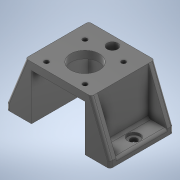
# Autodesk Inventor part: zmotorsupport
Saved by Autodesk Inventor 2020.2 (Build 242310000, 310)
## iProperties
Created: 2020-07-31
Part Number: zmotorsupport
Material: Generic
Document SubType Name: Modeling
Designer: JK
Density: 1 g/cm^3
Appearance: Smooth - Black
Author: JK
Autodesk Inventor part; units mm, degrees
ref_plane "YZ Plane" through (0, 0, 0) normal (1, 0, 0) x (0, 1, 0)
ref_plane "XZ Plane" through (0, 0, 0) normal (0, 1, 0) x (-1, 0, 0)
ref_plane "XY Plane" through (0, 0, 0) normal (0, 0, 1) x (1, 0, 0)
sketch "Sketch1" plane through (0, 0, 0) normal (0, 1, 0) x (-1, 0, 0)
  circle A0 centre (0, 0) radius 11.5
  circle A1 centre (0, -22) radius 4.25
  line L0 (-21.5, 21.5) -> (21.5, 21.5)
  line L1 (21.5, 21.5) -> (21.5, -21.5)
  line L2 (21.5, -21.5) -> (-21.5, -21.5)
  line L3 (-21.5, -21.5) -> (-21.5, 21.5)
  line L4 (-21.5, 21.5) -> (21.5, -21.5) construction
  line L5 (21.5, 21.5) -> (-21.5, -21.5) construction
  line L6 (21.5, -21.5) -> (-21.5, -21.5)
  line L7 (-21.5, -21.5) -> (-21.5, -29.5)
  line L8 (-21.5, -29.5) -> (21.5, -29.5)
  line L9 (21.5, -29.5) -> (21.5, -21.5)
  circle A2 centre (15.5, 15.5) radius 1.8
  circle A3 centre (15.5, -15.5) radius 1.8
  circle A4 centre (-15.5, -15.5) radius 1.8
  circle A5 centre (-15.5, 15.5) radius 1.8
  point P0 (0, 0)
  dimension "d0" = 23
  dimension "d1" = 22
  dimension "d2" = 8.5
  dimension "d3" = 43
  dimension "d4" = 43
  dimension "d5" = 3.6
  dimension "d6" = 31
  dimension "d7" = 31
  dimension "d8" = 8
  constraints: 20 end point, 6 centre point, 4 parallel, 4 point on line, 3 equal radius, 3 midpoint, 2 horizontal, 2 horizontal alignment, 2 perpendicular, 2 vertical alignment, 1 coincident
  measures "d0" diameter of A0
  measures "d1" distance of A1.centre point (0, 0)
  measures "d2" diameter of A1
  measures "d3" distance of L0.start L0.end
  measures "d4" distance of L0.end L1.end
  measures "d5" diameter of A3
  measures "d6" distance of A2.centre A3.centre
  measures "d7" distance of A4.centre A3.centre
  measures "d8" distance of L8.end L1.end
extrude "Extrusion1" add sketch "Sketch1" along normal blind 6 contours A1 L2 L9 L8 L7 | A1 L2 L3 L0 L1
sketch "Sketch2" plane through (0, 6, 0) normal (0, 1, 0) x (1, 0, 0)
  line L0 (-21.5, 29.5) -> (-21.5, -21.5) projected
  line L1 (-21.5, -21.5) -> (-26.5, -21.5)
  line L2 (-26.5, -21.5) -> (-26.5, 29.5)
  line L3 (-26.5, 29.5) -> (-21.5, 29.5)
  line L4 (-21.5, 29.5) -> (-21.5, -21.5)
  line L5 (21.5, -21.5) -> (26.5, -21.5)
  line L6 (26.5, -21.5) -> (26.5, 29.5)
  line L7 (26.5, 29.5) -> (21.5, 29.5)
  line L8 (21.5, 29.5) -> (21.5, -21.5)
  line L9 (-26.5, 29.5) -> (26.5, 29.5)
  line L10 (26.5, 29.5) -> (26.5, 24.5)
  line L11 (26.5, 24.5) -> (-26.5, 24.5)
  line L12 (-26.5, 24.5) -> (-26.5, 29.5)
  circle A0 centre (0, 22) radius 4.25 projected
  line L13 (21.5, 29.5) -> (-21.5, 29.5) projected
  point P0 (0, 0)
  point P1 (-21.5, 24.5)
  point P2 (-3.4369, 24.5)
  point P3 (3.4369, 24.5)
  point P4 (21.5, 24.5)
  point P5 (21.5, 29.5)
  dimension "d11" = 5
  dimension "d12" = 5
  dimension "d13" = 5
  constraints: 24 end point, 6 parallel, 3 horizontal, 3 perpendicular, 1 collinear, 1 point on line
  measures "d11" distance between parallel lines of L0 L2
  measures "d12" distance between parallel lines of L8 L6
  measures "d13" distance between parallel lines of L9 L11
extrude "Extrusion2" add sketch "Sketch2" against normal blind 43.081 contours L9 L8 L11 A0 L0 | L0 L11 L2 L3 | L0 L1 L2 L11 | L7 L6 L11 L8 | L11 L6 L5 L8
sketch "Sketch4" plane through (0, -37.081, 0) normal (0, -1, 0) x (1, 0, 0)
  line L0 (-26.5, 21.5) -> (26.5, 21.5) projected
  line L1 (26.5, 21.5) -> (41.5, 21.5)
  line L2 (41.5, 21.5) -> (41.5, -29.5)
  line L3 (41.5, -29.5) -> (26.5, -29.5)
  line L4 (26.5, -29.5) -> (26.5, 21.5)
  line L5 (-26.5, -29.5) -> (-26.5, 21.5) projected
  line L6 (-26.5, 21.5) -> (-41.5, 21.5)
  line L7 (-41.5, 21.5) -> (-41.5, -29.5)
  line L8 (-41.5, -29.5) -> (-26.5, -29.5)
  line L9 (-26.5, -29.5) -> (-26.5, 21.5)
  line L10 (-26.5, -29.5) -> (26.5, -29.5) projected
  circle A0 centre (-34, -5.25) radius 2.75
  circle A1 centre (34, -5.25) radius 2.75
  point P0 (0, 0)
  point P1 (-26.5, -29.5)
  dimension "d21" = 15
  dimension "d22" = 5.5
  dimension "d23" = 15
  dimension "d24" = 7.5
  dimension "d25" = 7.5
  dimension "d29" = 26.75
  constraints: 16 end point, 4 parallel, 2 centre point, 2 horizontal, 2 perpendicular, 1 collinear, 1 equal radius, 1 horizontal alignment
  measures "d21" distance between parallel lines of L5 L7
  measures "d22" diameter of A0
  measures "d23" distance between parallel lines of L2 L4
  measures "d24" distance from line of L5 A0.centre
  measures "d25" distance from line of L4 A1.centre
  measures "d29" distance from line of L1 A1.centre
extrude "Extrusion3" add sketch "Sketch4" against normal blind 5 contours L5 L8 L7 L6 | L1 L2 L3 L4
sketch "Sketch5" plane through (0, -32.081, 0) normal (0, 1, 0) x (1, 0, 0)
  circle A0 centre (-34, 5.25) radius 2.75 projected
  circle A1 centre (-34, 5.25) radius 5
  circle A2 centre (34, 5.25) radius 2.75 projected
  circle A3 centre (34, 5.25) radius 5
  point P0 (0, 0)
  dimension "d30" = 10
  constraints: 2 centre point, 2 coincident, 1 equal radius
  measures "d30" diameter of A1
extrude "Extrusion4" cut sketch "Sketch5" against normal blind 2 contours A1 | A2 | A3
sketch "Sketch7" plane through (26.5, 6, -29.5) normal (0, 0, -1) x (-1, 0, 0)
  line L0 (53, 0) -> (0, 0) projected
  line L1 (-15, -43.081) -> (-15, -38.081) projected
  line L2 (0, 0) -> (-15, -38.081)
  line L3 (-15, -38.081) -> (0, -38.081)
  line L4 (0, 0) -> (0, -38.081) projected
  line L5 (0, -38.081) -> (0, 0)
  line L6 (53, 0) -> (53, -38.081) projected
  line L7 (53, 0) -> (53, -38.081)
  line L8 (68, -38.081) -> (53, -38.081) projected
  line L9 (53, -38.081) -> (68, -38.081)
  line L10 (68, -38.081) -> (53, 0)
  point P0 (26.5, -6)
  constraints: 12 end point, 3 perpendicular, 1 collinear
extrude "Extrusion5" add sketch "Sketch7" against normal blind 5
sketch "Sketch8" plane through (-21.5, 0, 21.5) normal (0, 0, 1) x (1, 0, 0)
  line L0 (-5, -32.081) -> (-20, -32.081) projected
  line L1 (-5, 6) -> (-5, -32.081) projected
  line L2 (-5, 6) -> (-20, -32.081) projected
  line L3 (63, -32.081) -> (48, -32.081) projected
  line L4 (63, -32.081) -> (48, 6) projected
  line L5 (48, -32.081) -> (48, 6) projected
  point P0 (21.5, 0)
extrude "Extrusion6" add sketch "Sketch8" against normal blind 5
fillet "Fillet1" radius 2 4 edges at (41.5, -32.081, -4) (-41.5, -32.081, -4) (-26.5, -32.081, -4) (26.5, -32.081, -4)
fillet "Fillet2" radius 2 8 edges at (-41.5, -34.581, 21.5) (-41.5, -34.581, -29.5) (41.5, -34.581, 21.5) (41.5, -34.581, -29.5) (34, -13.0405, 21.5) (34, -13.0405, -29.5) (-34, -13.0405, 21.5) (-34, -13.0405, -29.5)
sketch "Sketch10" plane through (0, -37.081, 0) normal (0, -1, 0) x (1, 0, 0)
  line L0 (-46.933, 35.2152) -> (46.933, 35.2152)
  line L1 (46.933, 35.2152) -> (46.933, -35.2152)
  line L2 (46.933, -35.2152) -> (-46.933, -35.2152)
  line L3 (-46.933, -35.2152) -> (-46.933, 35.2152)
  line L4 (-46.933, 35.2152) -> (46.933, -35.2152) construction
  line L5 (46.933, 35.2152) -> (-46.933, -35.2152) construction
  point P0 (0, 0)
  constraints: 12 end point, 2 midpoint, 2 parallel, 1 horizontal, 1 perpendicular
sketch "Sketch9" plane through (0, 5, 0) normal (0, 1, 0) x (1, 0, 0)
  line L0 (41, 29) -> (41, -71) projected
  line L1 (41, 29) -> (-55.9789, 29)
  line L2 (-55.9789, 29) -> (-55.9789, -21)
  line L3 (-55.9789, -21) -> (41, -21)
  line L4 (41, -21) -> (41, 29)
  point P0 (0, 0)
  point P1 (41, -21)
  constraints: 8 end point, 2 parallel, 1 horizontal, 1 perpendicular
body "Solid1"
